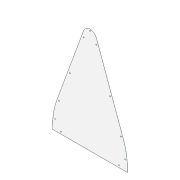
# Autodesk Inventor part: DBP-1-cover
Saved by Autodesk Inventor 2020 (Build 240168000, 168)
## iProperties
Created: 2021-06-21
Part Number: DBP-1-cover
Material: Generic
Document SubType Name: Modeling
Designer: Aidan Lee
Density: 1 g/cm^3
Appearance: Clear
Author: Aidan Lee
Autodesk Inventor part; units mm, degrees
ref_plane "YZ Plane" through (0, 0, 0) normal (1, 0, 0) x (0, 1, 0)
ref_plane "XZ Plane" through (0, 0, 0) normal (0, 1, 0) x (-1, 0, 0)
ref_plane "XY Plane" through (0, 0, 0) normal (0, 0, 1) x (1, 0, 0)
sketch "Sketch1" plane through (0, 0, 0) normal (0, 0, 1) x (1, 0, 0)
  line L0 (0, 0) -> (220, 0)
  line L1 (220, 0) -> (220, 10)
  line L2 (0, 10) -> (0, 0)
  line L3 (12.3995, 80.3208) -> (91.2061, 296.8404)
  circle A0 centre (110, 290) radius 11 construction
  line L4 (95.4021, 282.0544) -> (103.801, 305.1302) construction
  arc A1 (128.7939, 296.8404) -> (91.2061, 296.8404) centre (110, 290) ccw
  arc A2 (12.3995, 80.3208) -> (0, 10) centre (205.6042, 10) ccw
  line L5 (110, -51.553) -> (110, -95.4065)
  line L6 (207.6005, 80.3208) -> (128.7939, 296.8404)
  arc A3 (220, 10) -> (207.6005, 80.3208) centre (14.3958, 10) ccw
  line L7 (89.8628, 30.3395) -> (130.1372, 30.3395) construction
  line L8 (89.8628, 80.954) -> (130.1372, 80.954) construction
  line L9 (10, 0) -> (16, 0) construction
  line L10 (16, 0) -> (16, 25) construction
  line L11 (16, 25) -> (10, 25) construction
  line L12 (10, 25) -> (10, 0) construction
  line L13 (210, 0) -> (204, 0) construction
  line L14 (204, 0) -> (204, 25) construction
  line L15 (204, 25) -> (210, 25) construction
  line L16 (210, 25) -> (210, 0) construction
  line L17 (107, 0) -> (113, 0) construction
  line L18 (113, 0) -> (113, 25) construction
  line L19 (113, 25) -> (107, 25) construction
  line L20 (107, 25) -> (107, 0) construction
  spline S0 degree 5 poles (105.2685, 267.6918) (104.3685, 270.188) (101.9527, 273.6865) (95.9211, 275.1051) (84.9217, 261.7172) (84.2002, 254.5522) (73.4571, 234.9379) (71.7654, 203.3019) (99.8383, 234.2966) (104.2687, 244.3132) (107.1252, 256.6415) (106.5311, 264.1901) (105.2685, 267.6918) knots 0 0 0 0 0 0 0.117172 0.208109 0.323949 0.451788 0.587521 0.726569 0.835632 1 1 1 1 1 1 construction
  spline S1 degree 4 poles (110, 223.7331) (104.1843, 223.7331) (99.0728, 218.3206) (68.9468, 207.6663) (56.4589, 175.3769) (79.2984, 141.157) (95.289, 185.1681) (110, 185.1681) knots 0 0 0 0 0 0.26391 0.449807 0.665782 1 1 1 1 1 construction
  line L21 (105.419, 185.1681) -> (114.581, 185.1681) construction
  line L22 (106.6298, 223.7331) -> (113.3702, 223.7331) construction
  spline S2 degree 5 poles (61.2264, 152.1046) (56.7861, 151.4059) (49.5867, 147.2341) (40.4712, 132.1059) (34.2348, 112.2076) (27.9372, 89.519) (40.6073, 60.8371) (90.5177, 88.5345) (100.0799, 90.6107) (101.5037, 122.3299) (87.7725, 139.0296) (80.3941, 145.1495) (71.1893, 151.5941) (64.8383, 152.6729) (61.2264, 152.1046) knots 0 0 0 0 0 0 0.12324 0.20525 0.315018 0.423707 0.530897 0.635761 0.737213 0.827446 0.899752 1 1 1 1 1 1 construction
  spline S3 degree 5 poles (158.7736, 152.1046) (163.2139, 151.4059) (170.4133, 147.2341) (179.5288, 132.1059) (185.7652, 112.2076) (192.0628, 89.519) (179.3927, 60.8371) (129.4823, 88.5345) (119.9201, 90.6107) (118.4963, 122.3299) (132.2275, 139.0296) (139.6059, 145.1495) (148.8107, 151.5941) (155.1617, 152.6729) (158.7736, 152.1046) knots 0 0 0 0 0 0 0.12324 0.20525 0.315018 0.423707 0.530897 0.635761 0.737213 0.827446 0.899752 1 1 1 1 1 1 construction
  spline S4 degree 4 poles (110, 30.3395) (99.5705, 30.3395) (81.3994, 34.3322) (66.2735, 66.1691) (85.3554, 79.9322) (101.4268, 80.954) (110, 80.954) knots 0 0 0 0 0 0.389292 0.639292 1 1 1 1 1 construction
  spline S5 degree 4 poles (110, 30.3395) (120.4295, 30.3395) (138.6006, 34.3322) (153.7265, 66.1691) (134.6446, 79.9322) (118.5732, 80.954) (110, 80.954) knots 0 0 0 0 0 0.389292 0.639292 1 1 1 1 1 construction
  circle A4 centre (110, 290) radius 271 construction
  spline S6 degree 5 poles (22.7422, 63.6489) (18.8598, 60.4372) (14.7285, 50.7544) (16.9139, 26.9049) (28.0703, 17.1973) (49.017, 5.77) (101.1456, 4.5306) (84.8139, 28.9584) (61.4114, 52.3493) (50.7951, 59.5741) (34.6522, 68.0096) (26.4086, 66.6818) (22.7422, 63.6489) knots 0 0 0 0 0 0 0.151426 0.256435 0.381603 0.509507 0.638194 0.762008 0.856999 1 1 1 1 1 1 construction
  spline S7 degree 5 poles (197.2578, 63.6489) (201.1402, 60.4372) (205.2715, 50.7544) (203.0861, 26.9049) (191.9297, 17.1973) (170.983, 5.77) (118.8544, 4.5306) (135.1861, 28.9584) (158.5886, 52.3493) (169.2049, 59.5741) (185.3478, 68.0096) (193.5914, 66.6818) (197.2578, 63.6489) knots 0 0 0 0 0 0 0.151426 0.256435 0.381603 0.509507 0.638194 0.762008 0.856999 1 1 1 1 1 1 construction
  spline S8 degree 5 poles (114.7315, 267.6918) (115.6315, 270.188) (118.0473, 273.6865) (124.0789, 275.1051) (135.0783, 261.7172) (135.7998, 254.5522) (146.5429, 234.9379) (148.2346, 203.3019) (120.1617, 234.2966) (115.7313, 244.3132) (112.8748, 256.6415) (113.4689, 264.1901) (114.7315, 267.6918) knots 0 0 0 0 0 0 0.117172 0.208109 0.323949 0.451788 0.587521 0.726569 0.835632 1 1 1 1 1 1 construction
  line L23 (89.8628, 131.829) -> (130.1372, 131.829) construction
  line L24 (89.8628, 169.0772) -> (130.1372, 169.0772) construction
  spline S9 degree 4 poles (110, 169.0772) (104.4193, 169.0772) (95.377, 164.1793) (89.8577, 149.1245) (97.6407, 139.6025) (104.4855, 131.829) (110, 131.829) knots 0 0 0 0 0 0.377904 0.627904 1 1 1 1 1 construction
  spline S10 degree 4 poles (110, 169.0772) (115.5807, 169.0772) (124.623, 164.1793) (130.1423, 149.1245) (122.3593, 139.6025) (115.5145, 131.829) (110, 131.829) knots 0 0 0 0 0 0.377904 0.627904 1 1 1 1 1 construction
  spline S11 degree 4 poles (79.9792, 208.8227) (83.0253, 210.8992) (90.3751, 207.7383) (91.1743, 200.9673) (95.925, 189.2461) (95.6614, 183.9886) (95.7276, 177.0984) (93.3089, 174.5423) knots 0 0 0 0 0 0.301349 0.499604 0.699762 1 1 1 1 1 construction
  spline S12 degree 4 poles (99.1347, 219.9151) (96.3536, 218.4058) (93.9069, 213.4715) (95.6323, 204.9097) (99.5449, 192.6576) (102.4128, 188.2227) (107.1154, 185.1681) (110, 185.1681) knots 0 0 0 0 0 0.307399 0.5109 0.714193 1 1 1 1 1 construction
  spline S13 degree 4 poles (110, 223.7331) (115.8157, 223.7331) (120.9272, 218.3206) (151.0532, 207.6663) (163.5411, 175.3769) (140.7016, 141.157) (124.711, 185.1681) (110, 185.1681) knots 0 0 0 0 0 0.26391 0.449807 0.665782 1 1 1 1 1 construction
  spline S14 degree 4 poles (140.0208, 208.8227) (131.9358, 211.2642) (128.6549, 201.132) (123.2328, 188.7305) (123.9701, 180.7974) (126.6911, 174.5423) knots 0 0 0 0 0 0.499604 1 1 1 1 1 construction
  spline S15 degree 4 poles (120.8653, 219.9151) (125.9638, 216.9813) (125.7019, 209.3287) (121.6722, 194.6757) (117.597, 188.214) (112.8846, 185.1681) (110, 185.1681) knots 0 0 0 0 0 0.5109 0.714193 1 1 1 1 1 construction
  circle A5 centre (91.2791, 279.4979) radius 1.5
  circle A6 centre (110, 233.5775) radius 1.5 construction
  circle A7 centre (110, 103.2167) radius 1.5 construction
  circle A8 centre (24.6984, 6) radius 1.5
  circle A9 centre (19.3332, 81.8284) radius 1.5
  circle A10 centre (50.8614, 168.4513) radius 1.5
  circle A11 centre (128.7209, 279.4979) radius 1.5
  circle A12 centre (110, 233.5775) radius 1.5 construction
  circle A13 centre (110, 103.2167) radius 1.5 construction
  circle A14 centre (195.3016, 6) radius 1.5
  circle A15 centre (200.6668, 81.8284) radius 1.5
  circle A16 centre (169.1386, 168.4513) radius 1.5
  circle A17 centre (110, 305.5) radius 1.5
  line L25 (110, 305.5) -> (110, 301) construction
  line L26 (110, 305.5) -> (110, 310) construction
  circle A18 centre (6.9791, 29.7459) radius 1.5
  circle A19 centre (213.0209, 29.7459) radius 1.5
  line L27 (6.9791, 29.7459) -> (1.0085, 30.3395) construction
  line L28 (7.2595, 32.5665) -> (6.6987, 26.9254) construction
  line L29 (19.3332, 81.8284) -> (13.6951, 83.8805) construction
  line L30 (24.6984, 6) -> (24.6984, 0) construction
  line L31 (50.8614, 168.4513) -> (45.2233, 170.5035) construction
  line L32 (91.2791, 279.4979) -> (85.6409, 281.5501) construction
  point P0 (110, 0)
  point P1 (110, -73.4798)
  point P2 (110, 25)
  point P3 (89.6738, 266.316)
  point P4 (77.923, 217.7696)
  point P5 (95.4021, 231.2489)
  point P6 (99.0044, 219.8443)
  point P7 (73.6304, 203.8364)
  point P8 (64.1644, 177.5166)
  point P9 (76.0997, 161.4095)
  point P10 (35.1113, 113.8824)
  point P11 (32.4879, 90.0294)
  point P12 (45.995, 74.5523)
  point P13 (86.4381, 86.006)
  point P14 (98.1651, 99.0364)
  point P15 (96.7009, 123.3463)
  point P16 (86.4381, 139.2996)
  point P17 (75.5957, 148.0812)
  point P18 (184.8887, 113.8824)
  point P19 (187.5121, 90.0294)
  point P20 (174.005, 74.5523)
  point P21 (133.5619, 86.006)
  point P22 (121.8349, 99.0364)
  point P23 (123.2991, 123.3463)
  point P24 (133.5619, 139.2996)
  point P25 (144.4043, 148.0812)
  point P26 (83.1175, 40.7351)
  point P27 (75.5957, 63.6489)
  point P28 (86.4381, 76.9539)
  point P29 (136.8825, 40.7351)
  point P30 (144.4043, 63.6489)
  point P31 (133.5619, 76.9539)
  point P32 (28.2478, 19)
  point P33 (54.1698, 8.5933)
  point P34 (86.4381, 12.5)
  point P35 (83.1175, 28.0491)
  point P36 (61.2264, 51.1164)
  point P37 (41.4146, 63.6489)
  point P38 (191.7522, 19)
  point P39 (165.8302, 8.5933)
  point P40 (133.5619, 12.5)
  point P41 (136.8825, 28.0491)
  point P42 (158.7736, 51.1164)
  point P43 (178.5854, 63.6489)
  point P44 (76.1146, 233.5775)
  point P45 (83.6171, 255.3919)
  point P46 (105.324, 251.1657)
  point P47 (130.3262, 266.316)
  point P48 (142.077, 217.7696)
  point P49 (124.5979, 231.2489)
  point P50 (143.8854, 233.5775)
  point P51 (136.3829, 255.3919)
  point P52 (114.676, 251.1657)
  point P53 (96.9167, 162.2627)
  point P54 (93.4016, 150.3152)
  point P55 (98.1651, 139.607)
  point P56 (123.0833, 162.2627)
  point P57 (126.5984, 150.3152)
  point P58 (121.8349, 139.607)
  point P59 (88.2969, 207.1592)
  point P60 (92.0983, 199.5692)
  point P61 (94.8111, 190.7059)
  point P62 (95.6324, 183.3848)
  point P63 (95.1996, 213.8268)
  point P64 (96.2705, 203.5876)
  point P65 (99.6164, 193.7355)
  point P66 (103.463, 188.1501)
  point P67 (120.9956, 219.8443)
  point P68 (146.3696, 203.8364)
  point P69 (155.8356, 177.5166)
  point P70 (143.9003, 161.4095)
  point P71 (131.7031, 207.1592)
  point P72 (127.9017, 199.5692)
  point P73 (125.1889, 190.7059)
  point P74 (124.3676, 183.3848)
  point P75 (124.8004, 213.8268)
  point P76 (123.7295, 203.5876)
  point P77 (120.3836, 193.7355)
  point P78 (116.537, 188.1501)
  point P79 (120.8653, 219.9151)
  point P80 (126.6911, 174.5423)
  point P81 (140.0208, 208.8227)
  point P82 (124.5979, 282.0544)
  dimension "d2" = 22
  dimension "d1" = 220
  dimension "d4" = 9
  dimension "d7" = 290
  dimension "d8" = 20
  dimension "d9" = 10
  dimension "d10" = 25
  dimension "d11" = 6
  dimension "d12" = 542
  dimension "d19" = 10
  dimension "d35" = 3
  dimension "d38" = 6
  constraints: 66 end point, 61 symmetric about line, 24 horizontal, 19 centre point, 13 vertical alignment, 10 midpoint, 8 perpendicular, 8 point on circle, 7 equal length, 7 equal radius, 6 parallel, 6 point on line, 4 tangent, 2 coincident, 2 vertical, 1 collinear, 1 line through centre, 135 other
  measures "d1" distance of L0.start L0.end
  measures "d4" distance between parallel lines of L3 L4
  measures "d7" distance from line of L0 point (110, 290)
  measures "d8" angle of L2 L3
  measures "d9" distance from line of L2.start L0
  measures "d10" distance of L11.end L9.start
  measures "d11" distance between parallel lines of L10 L12
  measures "d12" diameter of A4
  measures "d19" distance from line of L12 L0.start
  measures "d35" diameter of A5
  measures "d38" distance from line of L27.end L28
extrude "Extrusion6" add sketch "Sketch1" along normal blind 0.5
body "Solid4"
